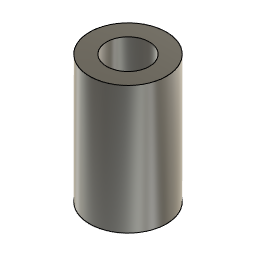
CepZaJednuStranuSipkeZaBilijar v1 (Autodesk Fusion 360 design; units mm, degrees)
Autodesk Fusion 360 part; units mm, degrees
sketch "Sketch1" plane through (0, 0, 0) normal (0, 0, 1) x (1, 0, 0)
  circle A0 centre (25, 25) radius 2.5
  circle A1 centre (25, 25) radius 4.5
  dimension "d1" = 5
  dimension "d2" = 9
  constraint concentric A0 A1
  measures "d1" diameter of A0
  measures "d2" diameter of A1
extrude "Extrude1" add sketch "Sketch1" along normal blind 10 contours A0 | A1
sketch "Sketch2" plane through (0, 0, 10) normal (0, 0, 1) x (-1, 0, 0)
  circle A0 centre (-25, -25) radius 4.5
extrude "Extrude2" add sketch "Sketch2" along normal blind 5
sketch "Sketch3" plane through (0, 0, 15) normal (0, 0, 1) x (-1, 0, 0)
  circle A0 centre (-25, -25) radius 4.5
  circle A1 centre (-25, -25) radius 2.5
  dimension "d7" = 5
  constraint concentric A0 A1
  measures "d7" diameter of A1
extrude "Extrude3" cut sketch "Sketch3" against normal blind 12 contours A1
